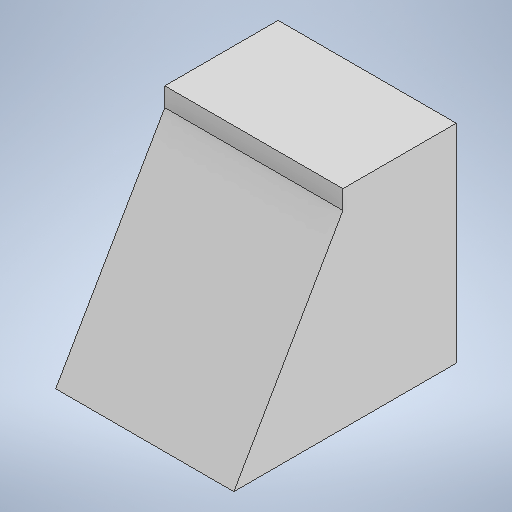
# Autodesk Inventor part: Side near railing 7
Saved by Autodesk Inventor 2025 (Build 290162000, 162)
## iProperties
Created: 2024-07-15
Part Number: Side near railing 7
Material: Generic
Document SubType Name: Modeling
Designer: track
Density: 1 g/cm^3
Appearance: Default
Author: track
Autodesk Inventor part; units mm, degrees
ref_plane "YZ Plane" through (0, 0, 0) normal (1, 0, 0) x (0, 1, 0)
ref_plane "XZ Plane" through (0, 0, 0) normal (0, 1, 0) x (-1, 0, 0)
ref_plane "XY Plane" through (0, 0, 0) normal (0, 0, 1) x (1, 0, 0)
sketch "Sketch1" plane through (0, 0, 0) normal (0, 1, 0) x (-1, 0, 0)
  line L0 (-838.2, 533.4) -> (838.2, 533.4)
  line L1 (838.2, 533.4) -> (838.2, -533.4)
  line L2 (838.2, -533.4) -> (-838.2, -533.4)
  line L3 (-838.2, -533.4) -> (-838.2, 533.4)
  line L4 (-838.2, 533.4) -> (838.2, -533.4) construction
  line L5 (838.2, 533.4) -> (-838.2, -533.4) construction
  point P0 (0, 0)
  dimension "d0" = 1676.4
  dimension "d1" = 1066.8
  constraints: 12 end point, 2 midpoint, 2 parallel, 1 horizontal, 1 perpendicular
  measures "d0" distance of L1.end L2.end
  measures "d1" distance of L2.end L0.start
extrude "Extrusion1" add sketch "Sketch1" against normal blind 1955.8
sketch "Sketch2" plane through (838.2, 0, 533.4) normal (1, 0, 0) x (0, 0, -1)
  line L0 (0, 0) -> (0, -1955.8) projected
  line L1 (0, -177.8) -> (0, -1955.8)
  line L2 (0, -1955.8) -> (-1026.5288, -1955.8)
  line L3 (-1026.5288, -1955.8) -> (0, -177.8)
  line L4 (0, 0) -> (1066.8, 0) projected
  point P0 (533.4, 0)
  dimension "d4" = 30
  dimension "d5" = 177.8
  constraints: 6 end point, 1 horizontal, 1 point on line, 1 vertical
  measures "d4" angle of L0 L3
  measures "d5" distance from line of L4 L1.start
extrude "Extrusion2" add sketch "Sketch2" against normal up to surface (1676.4 mm away)
body "Solid1"
